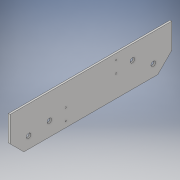
# Autodesk Inventor part: DriveTrain3.0
Saved by Autodesk Inventor 2017 (Build 210142000, 142)
## iProperties
Created: 2017-07-22
Part Number: DriveTrain3.0
Material: Generic
Document SubType Name: Modeling
Designer: User
Density: 1 g/cm^3
Appearance: Default
Author: User
Autodesk Inventor part; units mm, degrees
ref_plane "YZ Plane" through (0, 0, 0) normal (1, 0, 0) x (0, 1, 0)
ref_plane "XZ Plane" through (0, 0, 0) normal (0, 1, 0) x (-1, 0, 0)
ref_plane "XY Plane" through (0, 0, 0) normal (0, 0, 1) x (1, 0, 0)
sketch "Sketch1" plane through (0, 0, 0) normal (1, 0, 0) x (0, 1, 0)
  line L0 (0, 0) -> (107.95, 0)
  line L1 (107.95, 0) -> (107.95, -444.5)
  line L2 (107.95, -444.5) -> (0, -444.5)
  line L3 (0, -444.5) -> (0, 0)
  circle A0 centre (31.75, -50.8) radius 6.3627
  circle A1 centre (31.75, -393.7) radius 6.3627
  circle A2 centre (92.6338, -165.5318) radius 1.5875
  circle A3 centre (76.6318, -165.5318) radius 1.5875
  circle A4 centre (15.3162, -278.9682) radius 1.5875
  circle A5 centre (31.3182, -278.9682) radius 1.5875
  dimension "d0" = 107.95
  dimension "d1" = 444.5
  dimension "d2" = 12.7254
  dimension "d3" = 31.75
  dimension "d4" = 50.8
  dimension "d5" = 50.8
  dimension "d22" = 165.5318
  dimension "d23" = 3.175
  dimension "d24" = 15.3162
  dimension "d25" = 3.175
  dimension "d26" = 16.002
  dimension "d27" = 165.5318
  dimension "d28" = 3.175
  dimension "d29" = 15.3162
  dimension "d30" = 165.5318
  dimension "d31" = 3.175
  dimension "d32" = 16.002
  dimension "d33" = 165.5318
  constraints: 8 end point, 6 centre point, 2 parallel, 1 horizontal, 1 perpendicular
  measures "d0" distance of L1.end L2.end
  measures "d1" distance of L0.end L1.end
  measures "d2" diameter of A0
  measures "d3" distance from line of L3 A0.centre
  measures "d4" distance from line of L0 A0.centre
  measures "d5" distance from line of L2 A1.centre
  measures "d22" distance from line of L0 A2.centre
  measures "d23" diameter of A2
  measures "d24" distance from line of L1 A2.centre
  measures "d25" diameter of A3
  measures "d26" distance of A2.centre A3.centre
  measures "d27" distance from line of L0 A3.centre
  measures "d28" diameter of A4
  measures "d29" distance from line of L3 A4.centre
  measures "d30" distance from line of L2 A4.centre
  measures "d31" diameter of A5
  measures "d32" distance of A5.centre A4.centre
  measures "d33" distance from line of L2 A5.centre
extrude "Extrusion1" add sketch "Sketch1" along normal blind 4.7625 contours L0 L1 L2 L3 | A2 | A3 | A4 | A5
chamfer "Chamfer1" distance 38.1 angle 45 1 edges at (2.3813, 0, 0)
chamfer "Chamfer2" distance 38.1 angle 45 1 edges at (2.3813, 0, -444.5)
sketch "Sketch2" plane through (4.7625, 0, 0) normal (1, 0, 0) x (0, 0, -1)
  line L0 (444.5, 38.1) -> (406.4, 0) projected
  line L1 (444.5, 38.1) -> (444.5, 107.95) projected
  line L2 (444.5, 107.95) -> (0, 107.95) projected
  line L3 (0, 107.95) -> (0, 38.1) projected
  line L4 (38.1, 0) -> (0, 38.1) projected
  line L5 (38.1, 0) -> (406.4, 0) projected
  circle A0 centre (393.7, 31.75) radius 6.3627 projected
  circle A1 centre (50.8, 31.75) radius 6.3627 projected
  circle A2 centre (107.95, 38.989) radius 6.3627
  circle A3 centre (336.55, 68.961) radius 6.3627
  point P0 (0, 0)
  dimension "d14" = 12.7254
  dimension "d15" = 107.95
  dimension "d17" = 12.7254
  dimension "d19" = 107.95
  dimension "d78" = 38.989
  dimension "d79" = 38.989
  constraints: 2 centre point
  measures "d14" diameter of A2
  measures "d15" distance from line of L3 A2.centre
  measures "d17" diameter of A3
  measures "d19" distance from line of L1 A3.centre
  measures "d78" distance from line of L5 A2.centre
  measures "d79" distance from line of L2 A3.centre
extrude "Extrusion2" cut sketch "Sketch2" against normal blind 25.4 contours A2 | A3
sketch "Sketch6" plane through (4.7625, 0, 0) normal (1, 0, 0) x (0, 0, -1)
  circle A0 centre (107.95, 38.989) radius 6.3627 projected
  circle A1 centre (336.55, 68.961) radius 6.3627 projected
  line L0 (444.5, 38.1) -> (406.4, 0) projected
  line L1 (444.5, 38.1) -> (444.5, 107.95) projected
  line L2 (444.5, 107.95) -> (0, 107.95) projected
  line L3 (0, 107.95) -> (0, 38.1) projected
  line L4 (38.1, 0) -> (0, 38.1) projected
  line L5 (38.1, 0) -> (406.4, 0) projected
  circle A2 centre (393.7, 31.75) radius 6.3627 projected
  circle A3 centre (50.8, 31.75) radius 6.3627 projected
  point P0 (0, 0)
  point P1 (153.0604, 48.006)
  point P2 (153.0604, 16.002)
  point P3 (291.4396, 91.948)
  point P4 (291.4396, 59.944)
  dimension "d80" = 32.004
  dimension "d81" = 45.1104
  dimension "d82" = 45.1104
  dimension "d83" = 16.002
  dimension "d84" = 45.1104
  dimension "d85" = 45.1104
  dimension "d86" = 32.004
  dimension "d87" = 16.002
  measures "d80" distance of point (153.06, 16.002) point (153.06, 48.006)
  measures "d81" horizontal distance of A0.centre point (153.06, 16.002)
  measures "d82" horizontal distance of A0.centre point (153.06, 48.006)
  measures "d83" distance from line of L5 point (153.06, 16.002)
  measures "d84" horizontal distance of A1.centre point (291.44, 59.944)
  measures "d85" horizontal distance of point (291.44, 91.948) A1.centre
  measures "d86" distance of point (291.44, 59.944) point (291.44, 91.948)
  measures "d87" distance from line of L2 point (291.44, 91.948)
hole "Hole1" at (4.7625, 48.006, -153.0604) at (4.7625, 16.002, -153.0604) at (4.7625, 91.948, -291.4396) at (4.7625, 59.944, -291.4396) direction (-1, 0, 0) diameter 3.81 end through all
equation "\"d82\" = d81"
body "Solid1"
